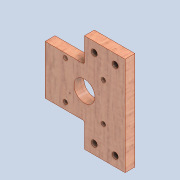
# Autodesk Inventor part: 0005-10-023 Suport motor x
Saved by Autodesk Inventor 2020 (Build 240168000, 168)
## iProperties
Created: 2020-12-18
Part Number: 0005-10-023 Suport motor x
Material: Wood (Maple)
Document SubType Name: Modeling
Designer: Iulian Bors
Density: 0.67 g/cm^3
Appearance: White Oak - Natural Medium Gloss
Mass: 19.1673 g
Surface Area: 107.538 cm^2
Volume: 28.608 cm^3
Author: Iulian Bors
Subject: 023
Autodesk Inventor part; units mm, degrees
ref_plane "YZ Plane" through (0, 0, 0) normal (1, 0, 0) x (0, 1, 0)
ref_plane "XZ Plane" through (0, 0, 0) normal (0, 1, 0) x (-1, 0, 0)
ref_plane "XY Plane" through (0, 0, 0) normal (0, 0, 1) x (1, 0, 0)
sketch "Sketch1" plane through (0, 0, 0) normal (0, 0, 1) x (1, 0, 0)
  line L0 (-32.5, 20) -> (32.5, 20)
  line L1 (32.5, 20) -> (32.5, -20)
  line L2 (32.5, -20) -> (-32.5, -20)
  line L3 (-32.5, -20) -> (-32.5, 20)
  point P0 (0, 0)
  point P1 (0, 20)
  point P2 (-32.5, 0)
  dimension "d0" = 65
  dimension "d1" = 40
  constraints: 8 end point, 2 midpoint, 2 parallel, 1 horizontal, 1 horizontal alignment, 1 perpendicular, 1 vertical alignment
  measures "d0" distance of L0.start L0.end
  measures "d1" distance of L2.end L0.start
extrude "Extrusion1" add sketch "Sketch1" along normal blind 8
sketch "Sketch5" plane through (0, 0, 0) normal (0, 0, -1) x (-1, 0, 0)
  line L0 (-32.5, 40) -> (0.5, 40)
  line L1 (0.5, 40) -> (0.5, -40)
  line L2 (0.5, -40) -> (-32.5, -40)
  line L3 (-32.5, -40) -> (-32.5, 40)
  line L4 (-32.5, -20) -> (-32.5, 20) projected
  line L5 (-32.5, 20) -> (32.5, 20) projected
  line L6 (32.5, -20) -> (-32.5, -20) projected
  point P0 (0, 0)
  dimension "d22" = 20
  dimension "d23" = 20
  dimension "d24" = 33
  constraints: 8 end point, 2 parallel, 1 collinear, 1 horizontal, 1 perpendicular
  measures "d22" distance between parallel lines of L5 L0
  measures "d23" distance between parallel lines of L2 L6
  measures "d24" distance between parallel lines of L3 L1
extrude "Extrusion5" add sketch "Sketch5" against normal up to surface (8 mm away)
sketch "Sketch6" plane through (0, 0, 0) normal (0, 0, -1) x (-1, 0, 0)
  line L0 (0.5, 40) -> (-32.5, 40) projected
  line L1 (-32.5, 40) -> (-32.5, -40) projected
  line L2 (-15, 16.5) -> (16, 16.5) construction
  line L3 (16, 16.5) -> (16, -14.5) construction
  line L4 (16, -14.5) -> (-15, -14.5) construction
  line L5 (-15, -14.5) -> (-15, 16.5) construction
  line L6 (-15, 16.5) -> (16, -14.5) construction
  line L7 (16, 16.5) -> (-15, -14.5) construction
  circle A0 centre (-15, 16.5) radius 1.75
  circle A1 centre (16, 16.5) radius 1.75
  circle A2 centre (16, -14.5) radius 1.75
  circle A3 centre (-15, -14.5) radius 1.75
  circle A4 centre (0.5, 1) radius 8.5
  dimension "d29" = 31
  dimension "d30" = 33
  dimension "d31" = 39
  dimension "d32" = 3.5
  dimension "d33" = 17
  constraints: 12 end point, 5 centre point, 4 coincident, 3 equal radius, 2 midpoint, 2 parallel, 2 perpendicular, 1 horizontal
  measures "d29" distance of L2.start L2.end
  measures "d30" distance from line of L1 point (0.5, 1)
  measures "d31" distance from line of point (0.5, 1) L0
  measures "d32" diameter of A0
  measures "d33" diameter of A4
extrude "Extrusion6" cut sketch "Sketch6" against normal blind 10
sketch "Sketch7" plane through (0, 0, 0) normal (0, 0, -1) x (-1, 0, 0)
  line L0 (-32.5, 40) -> (-32.5, -40) projected
  line L1 (0.5, 40) -> (-32.5, 40) projected
  line L2 (0.5, 20) -> (0.5, 40) projected
  line L3 (-32.5, -40) -> (0.5, -40) projected
  point P0 (0, 0)
  point P1 (-24.5, 32)
  point P2 (-7.5, 32)
  point P3 (-24.5, -32)
  point P4 (-7.5, -32)
  dimension "d36" = 8
  dimension "d37" = 8
  dimension "d38" = 8
  dimension "d39" = 17
  dimension "d40" = 8
  dimension "d41" = 64
  constraints: 2 horizontal alignment, 2 vertical alignment
  measures "d36" distance from line of L0 point (-24.5, 32)
  measures "d37" distance from line of point (-24.5, 32) L1
  measures "d38" distance from line of L2 point (-7.5, 32)
  measures "d39" distance of point (-7.5, 32) point (-24.5, 32)
  measures "d40" distance from line of L3 point (-24.5, -32)
  measures "d41" distance of point (-24.5, -32) point (-24.5, 32)
hole "Hole1" at (24.5, 32, 0) direction (0, 0, 1) diameter 5 end through all
pattern_linear "Rectangular Pattern1" count 2 spacing 64 along (0, -1, 0) count 2 spacing 17 along (-1, 0, 0) of "Hole1"
fillet "Fillet1" radius 1.5 2 edges at (-0.5, -20, 4) (-0.5, 20, 4)
equation "\"d23\" = d22"
equation "\"d38\" = d36"
equation "\"d40\" = d37"
body "Solid1"
